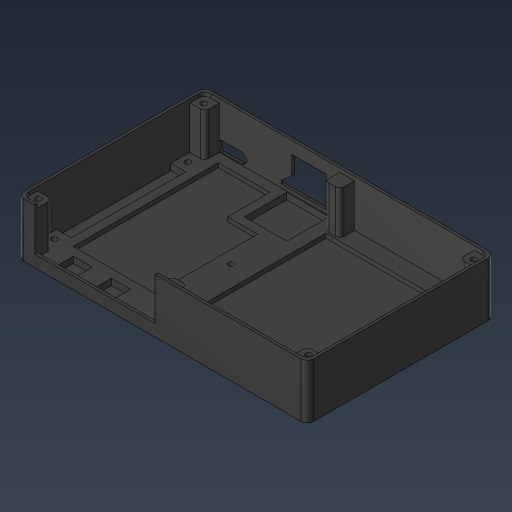
# Autodesk Inventor part: Gehaeuse BS v3
Saved by Autodesk Inventor 2023.1 (Build 271208000, 208)
## iProperties
Part Number: Gehaeuse BS v3
Material: PC/ABS-Kunststoff
Document SubType Name: Modeling
Designer: rYan
Density: 0.357273 g/cm^3
Appearance: Glatt - Schwarz
Mass: 15.1858 g
Surface Area: 455.446 cm^2
Volume: 42.5049 cm^3
Author: rYan
Autodesk Inventor part; units mm, degrees
ref_plane "YZ Plane" through (0, 0, 0) normal (1, 0, 0) x (0, 1, 0)
ref_plane "XZ Plane" through (0, 0, 0) normal (0, 1, 0) x (-1, 0, 0)
ref_plane "XY Plane" through (0, 0, 0) normal (0, 0, 1) x (1, 0, 0)
sketch "Skizze1" plane through (0, 0, 0) normal (0, 0, 1) x (1, 0, 0)
  line L0 (-68.45, -44.2) -> (68.45, -44.2)
  line L1 (68.45, -44.2) -> (68.45, 44.2)
  line L2 (68.45, 44.2) -> (-68.45, 44.2)
  line L3 (-68.45, 44.2) -> (-68.45, -44.2)
  line L4 (-68.45, -44.2) -> (68.45, 44.2) construction
  line L5 (68.45, -44.2) -> (-68.45, 44.2) construction
  circle A0 centre (-63.75, -39) radius 1.375
  circle A1 centre (63.75, -39) radius 1.375
  circle A2 centre (63.75, 39) radius 1.375
  circle A3 centre (-63.75, 39) radius 1.375
  line L6 (0, 61.88) -> (0, -61.88) projected
  line L7 (-95.83, 0) -> (95.83, 0) projected
  circle A4 centre (-63.75, 31.5) radius 1.375
  circle A5 centre (-63.75, -31.5) radius 1.375
  line L8 (-63.75, 39) -> (-63.75, 31.5) construction
  circle A6 centre (-11.75, 0) radius 1.375
  point P0 (0, 0)
  dimension "d0" = 136.9
  dimension "d1" = 88.4
  dimension "d2" = 2.75
  dimension "d3" = 127.5
  dimension "d4" = 78
  dimension "d7" = 63
  dimension "d8" = 2.75
  dimension "d9" = 2.75
  dimension "d10" = 52
  constraints: 14 end point, 7 centre point, 2 midpoint, 2 parallel, 1 horizontal, 1 perpendicular, 1 point on line, 1 vertical, 4 other
  measures "d0" distance of L2.end L1.end
  measures "d1" distance of L1.end L0.end
  measures "d2" diameter of A3
  measures "d3" distance of A1.centre A0.centre
  measures "d4" distance of A0.centre L8.start
  measures "d7" distance of A5.centre L8.end
  measures "d8" diameter of A4
  measures "d9" diameter of A6
  measures "d10" horizontal distance of A6.centre L8.end
extrude "Extrusion1" add sketch "Skizze1" along normal blind 3.6 contours L3 L7 A6 L6 L0 | L6 L7 L1 L0 | L3 L2 L6 L7 A6 | L6 L2 L1 L7
sketch "Skizze2" plane through (0, 0, 0) normal (0, 0, -1) x (-1, 0, 0)
  circle A0 centre (63.75, -31.5) radius 1.375 projected
  circle A1 centre (63.75, 31.5) radius 1.375 projected
  circle A2 centre (11.75, 0) radius 1.375 projected
  line L0 (67.05, -28.2) -> (60.45, -28.2)
  line L1 (60.45, -28.2) -> (60.45, -34.8)
  line L2 (60.45, -34.8) -> (67.05, -34.8)
  line L3 (67.05, -34.8) -> (67.05, -28.2)
  line L4 (67.05, -28.2) -> (60.45, -34.8) construction
  line L5 (60.45, -28.2) -> (67.05, -34.8) construction
  line L6 (67.05, 34.8) -> (60.45, 34.8)
  line L7 (60.45, 34.8) -> (60.45, 28.2)
  line L8 (60.45, 28.2) -> (67.05, 28.2)
  line L9 (67.05, 28.2) -> (67.05, 34.8)
  circle A3 centre (63.75, 31.5) radius 1.375 projected
  line L10 (67.05, 34.8) -> (60.45, 28.2) construction
  line L11 (60.45, 34.8) -> (67.05, 28.2) construction
  line L12 (15.05, 3.3) -> (8.45, 3.3)
  line L13 (8.45, 3.3) -> (8.45, -3.3)
  line L14 (8.45, -3.3) -> (15.05, -3.3)
  line L15 (15.05, -3.3) -> (15.05, 3.3)
  line L16 (15.05, 3.3) -> (8.45, -3.3) construction
  line L17 (8.45, 3.3) -> (15.05, -3.3) construction
  point P0 (0, 0)
  dimension "d11" = 6.6
  dimension "d12" = 6.6
  constraints: 36 end point, 6 midpoint, 6 parallel, 4 equal length, 3 horizontal, 3 perpendicular
  measures "d11" distance of L2.end L1.end
  measures "d12" distance of L1.end L0.end
extrude "Extrusion2" [suppressed]
sketch "Skizze3" plane through (0, 0, 3.6) normal (0, 0, 1) x (1, 0, 0)
  circle A0 centre (-63.75, 31.5) radius 1.375 projected
  circle A1 centre (-63.75, -31.5) radius 1.375 projected
  circle A2 centre (-11.75, 0) radius 1.375 projected
  line L0 (-63.75, 31.5) -> (-63.75, -31.5) construction
  line L1 (-95.83, 0) -> (95.83, 0) projected
  line L2 (-67.25, -27) -> (-60.25, -27)
  line L3 (-60.25, -27) -> (-60.25, 27)
  line L4 (-60.25, 27) -> (-67.25, 27)
  line L5 (-67.25, 27) -> (-67.25, -27)
  line L6 (-67.25, -27) -> (-60.25, 27) construction
  line L7 (-60.25, -27) -> (-67.25, 27) construction
  line L8 (-52.25, -34) -> (-43.25, -34)
  line L9 (-43.25, -34) -> (-43.25, -43)
  line L10 (-43.25, -43) -> (-52.25, -43)
  line L11 (-52.25, -43) -> (-52.25, -34)
  line L12 (-34.25, -34) -> (-25.25, -34)
  line L13 (-25.25, -34) -> (-25.25, -43)
  line L14 (-25.25, -43) -> (-34.25, -43)
  line L15 (-34.25, -43) -> (-34.25, -34)
  line L16 (-47.75, -34) -> (-47.75, -43) construction
  line L17 (-29.75, -34) -> (-29.75, -43) construction
  line L18 (-52.25, -38.5) -> (-43.25, -38.5) construction
  line L19 (-27.95, 22.5) -> (-7.95, 22.5)
  line L20 (-7.95, 22.5) -> (-7.95, 42.5)
  line L21 (-7.95, 42.5) -> (-27.95, 42.5)
  line L22 (-27.95, 42.5) -> (-27.95, 22.5)
  line L23 (-17.95, 42.5) -> (-17.95, 22.5) construction
  point P0 (0, 0)
  point P1 (-63.75, 0)
  dimension "d15" = 7
  dimension "d16" = 54
  dimension "d17" = 9
  dimension "d18" = 9
  dimension "d19" = 9
  dimension "d20" = 18
  dimension "d21" = 16
  dimension "d22" = 7
  dimension "d23" = 20
  dimension "d25" = 11
  dimension "d26" = 20
  dimension "d29" = 45.8
  constraints: 46 end point, 11 midpoint, 8 parallel, 4 horizontal, 4 perpendicular, 3 point on line, 1 vertical
  measures "d15" distance of L4.end L3.end
  measures "d16" distance of L3.end L2.end
  measures "d17" distance of L8.start L8.end
  measures "d18" distance of L12.start L12.end
  measures "d19" distance of L10.end L8.start
  measures "d20" distance between parallel lines of L17 L16
  measures "d21" distance between parallel lines of L16 L0
  measures "d22" distance from line of L18 L0.end
  measures "d23" distance of L19.start L19.end
  measures "d25" distance from line of L21 L0.start
  measures "d26" distance of L19.end L20.end
  measures "d29" distance between parallel lines of L23 L0
extrude "Extrusion3" cut sketch "Skizze3" against normal blind 3 contours L3 L2 L5 L1 | L1 L5 L4 L3 | L8 L9 L10 L11 | L12 L13 L14 L15 | L22 L21 L20 L19
sketch "Skizze4" plane through (0, 0, 3.6) normal (0, 0, 1) x (1, 0, 0)
  line L0 (-31.95, 18.5) -> (-17.75, 18.5)
  line L1 (-17.75, 18.5) -> (-17.75, -30)
  line L2 (-17.75, -30) -> (-56.25, -30)
  line L3 (-56.25, -30) -> (-56.25, 38.5)
  line L4 (-31.95, 18.5) -> (-31.95, 38.5)
  line L5 (-31.95, 38.5) -> (-56.25, 38.5)
  line L6 (-1.95, 35) -> (58.05, 35)
  line L7 (58.05, 35) -> (58.05, -35)
  line L8 (58.05, -35) -> (-1.95, -35)
  line L9 (-1.95, -35) -> (-1.95, 35)
  line L10 (-7.95, 22.5) -> (-27.95, 22.5) projected
  line L11 (-7.95, 42.5) -> (-7.95, 22.5) projected
  line L12 (-27.95, 42.5) -> (-7.95, 42.5) projected
  line L13 (-27.95, 22.5) -> (-27.95, 42.5) projected
  line L14 (-60.25, -27) -> (-67.25, -27) projected
  line L15 (-60.25, 27) -> (-60.25, -27) projected
  line L16 (-67.25, 27) -> (-60.25, 27) projected
  line L17 (-67.25, -27) -> (-67.25, 27) projected
  line L18 (-34.25, -34) -> (-25.25, -34) projected
  line L19 (-34.25, -43) -> (-34.25, -34) projected
  line L20 (-25.25, -43) -> (-34.25, -43) projected
  line L21 (-25.25, -34) -> (-25.25, -43) projected
  circle A0 centre (-11.75, 0) radius 1.375 projected
  line L22 (-95.83, 0) -> (95.83, 0) projected
  line L23 (0, 61.88) -> (0, -61.88) projected
  point P0 (0, 0)
  dimension "d30" = 4
  dimension "d31" = 4
  dimension "d32" = 4
  dimension "d34" = 4
  dimension "d35" = 6
  dimension "d36" = 4
  dimension "d37" = 6
  dimension "d38" = 70
  dimension "d39" = 60
  constraints: 20 end point, 4 parallel, 2 horizontal, 2 perpendicular, 1 other
  measures "d30" distance between parallel lines of L15 L3
  measures "d31" distance between parallel lines of L4 L13
  measures "d32" distance between parallel lines of L12 L5
  measures "d34" distance between parallel lines of L18 L2
  measures "d35" distance from line of L1 A0.centre
  measures "d36" distance between parallel lines of L10 L0
  measures "d37" distance between parallel lines of L11 L9
  measures "d38" distance of L6.end L7.end
  measures "d39" distance of L6.start L6.end
extrude "Extrusion4" cut sketch "Skizze4" against normal blind 2 contours L9 L6 L23 L22 | L22 L23 L8 L9 | L0 L1 L22 L3 L5 L4 | L1 L2 L3 L22 | L23 L6 L7 L22 | L22 L7 L8 L23
sketch "Skizze5" plane through (0, 0, 3.6) normal (0, 0, 1) x (1, 0, 0)
  circle A0 centre (-63.75, 39) radius 1.375 projected
  circle A1 centre (-63.75, -39) radius 1.375 projected
  circle A2 centre (63.75, -39) radius 1.375 projected
  circle A3 centre (63.75, 39) radius 1.375 projected
  line L0 (-67.25, 43) -> (-60.25, 43)
  line L1 (-60.25, 43) -> (-60.25, 36)
  line L2 (-60.25, 36) -> (-67.25, 36)
  line L3 (-67.25, 36) -> (-67.25, 43)
  line L4 (-67.25, -43) -> (-60.25, -43)
  line L5 (-60.25, -43) -> (-60.25, -36)
  line L6 (-60.25, -36) -> (-67.25, -36)
  line L7 (-67.25, -36) -> (-67.25, -43)
  line L8 (60.25, 36) -> (67.25, 36)
  line L9 (67.25, 36) -> (67.25, 43)
  line L10 (67.25, 43) -> (60.25, 43)
  line L11 (60.25, 43) -> (60.25, 36)
  circle A4 centre (63.75, 39) radius 1.375 projected
  line L12 (60.25, -43) -> (67.25, -43)
  line L13 (67.25, -43) -> (67.25, -36)
  line L14 (67.25, -36) -> (60.25, -36)
  line L15 (60.25, -36) -> (60.25, -43)
  line L16 (0, 61.88) -> (0, -61.88) projected
  line L17 (-95.83, 0) -> (95.83, 0) projected
  line L18 (-63.75, 36) -> (-63.75, 43) construction
  line L19 (3.5, -43) -> (-3.5, -43)
  line L20 (-3.5, -43) -> (-3.5, -36)
  line L21 (-3.5, -36) -> (3.5, -36)
  line L22 (3.5, -36) -> (3.5, -43)
  line L23 (3.5, 36) -> (-3.5, 36)
  line L24 (-3.5, 36) -> (-3.5, 43)
  line L25 (-3.5, 43) -> (3.5, 43)
  line L26 (3.5, 43) -> (3.5, 36)
  point P0 (0, 0)
  dimension "d42" = 7
  dimension "d46" = 3
  dimension "d47" = 4
  dimension "d51" = 7
  constraints: 50 end point, 12 parallel, 6 horizontal, 6 perpendicular, 4 collinear, 2 midpoint, 2 point on line, 14 other
  measures "d42" distance of L1.end L2.end
  measures "d46" distance from line of L2 A0.centre
  measures "d47" distance from line of L0 A0.centre
  measures "d51" distance of L19.start L19.end
extrude "Extrusion5" add sketch "Skizze5" along normal blind 20.2
sketch "Skizze7" plane through (0, 0, 23.8) normal (0, 0, 1) x (1, 0, 0)
  line L0 (-3.5, -43) -> (3.5, -43) projected
  line L1 (3.5, -43) -> (3.5, -36) projected
  line L2 (3.5, -36) -> (-3.5, -36) projected
  line L3 (-3.5, -36) -> (-3.5, -43) projected
  point P0 (0, 0)
extrude "Extrusion7" cut sketch "Skizze7" against normal blind 3.2
fillet "Rundung1" radius 2 8 edges at (-60.25, 36, 13.7) (-60.25, -36, 13.7) (60.25, 36, 13.7) (60.25, -36, 13.7) (3.5, -36, 12.1) (3.5, 36, 13.7) (-3.5, 36, 13.7) (-3.5, -36, 12.1)
sketch "Skizze6" plane through (0, 0, 3.6) normal (0, 0, 1) x (1, 0, 0)
  line L0 (-60.25, 43) -> (-67.25, 43) projected
  line L1 (-67.25, 43) -> (-67.25, 36) projected
  line L2 (67.25, -43) -> (67.25, -36) projected
  line L3 (60.25, -43) -> (67.25, -43) projected
  line L4 (-67.25, 43) -> (67.25, 43)
  line L5 (67.25, 43) -> (67.25, -43)
  line L6 (67.25, -43) -> (-67.25, -43)
  line L7 (-67.25, -43) -> (-67.25, 43)
  line L8 (68.45, 44.2) -> (-68.45, 44.2)
  line L9 (-68.45, 44.2) -> (-68.45, -44.2)
  line L10 (-68.45, -44.2) -> (68.45, -44.2)
  line L11 (68.45, -44.2) -> (68.45, 44.2)
  point P0 (0, 0)
  dimension "d48" = 1.2
  constraints: 16 end point, 4 parallel, 2 perpendicular, 1 horizontal, 3 other
  measures "d48" distance between parallel lines of L4 L8
extrude "Extrusion6" add sketch "Skizze6" along normal blind 22
sketch "Skizze8" plane through (-68.45, 44.2, 0) normal (0, 1, 0) x (1, 0, 0)
  line L0 (68.45, 3.96) -> (68.45, -23.76) projected
  line L1 (164.28, 0) -> (-27.38, 0) projected
  line L2 (19.2, -4) -> (8.2, -4)
  line L3 (8.2, -4) -> (8.2, -9)
  line L4 (8.2, -9) -> (19.2, -9)
  line L5 (19.2, -9) -> (19.2, -4)
  line L6 (19.2, -4) -> (8.2, -9) construction
  line L7 (8.2, -4) -> (19.2, -9) construction
  line L8 (58.55, -5.2) -> (42.35, -5.2)
  line L9 (42.35, -5.2) -> (42.35, -19.8)
  line L10 (42.35, -19.8) -> (58.55, -19.8)
  line L11 (58.55, -19.8) -> (58.55, -5.2)
  line L12 (58.55, -5.2) -> (42.35, -19.8) construction
  line L13 (42.35, -5.2) -> (58.55, -19.8) construction
  line L14 (42.35, -5.2) -> (37.35, -5.2)
  line L15 (37.35, -5.2) -> (37.35, -6.7)
  line L16 (37.35, -6.7) -> (42.35, -10.8955)
  line L17 (19.2, -9) -> (21.7, -6.5)
  line L18 (21.7, -6.5) -> (19.2, -4)
  line L19 (21.7, -6.5) -> (13.7, -6.5) construction
  point P0 (68.45, 0)
  point P1 (50.45, -12.5)
  dimension "d55" = 54.75
  dimension "d56" = 6.5
  dimension "d57" = 11
  dimension "d58" = 5
  dimension "d61" = 18
  dimension "d63" = 14.6
  dimension "d64" = 16.2
  dimension "d65" = 5.2
  dimension "d66" = 50
  dimension "d67" = 1.5
  dimension "d68" = 5
  dimension "d69" = 2.5
  constraints: 36 end point, 4 horizontal, 4 midpoint, 4 parallel, 3 perpendicular, 3 point on line, 1 vertical, 1 other
  measures "d55" distance from line of L0 L19.end
  measures "d56" distance from line of L1 L19.end
  measures "d57" distance of L3.end L4.end
  measures "d58" distance of L4.end L2.start
  measures "d61" distance from line of L0 point (50.45, -12.5)
  measures "d63" distance of L10.end L8.start
  measures "d64" distance of L9.end L10.end
  measures "d65" distance between parallel lines of L8 L1
  measures "d66" angle of L16 L15
  measures "d67" distance of L14.end L15.end
  measures "d68" distance of L8.end L14.end
  measures "d69" distance from line of L5 L17.end
extrude "Extrusion8" cut sketch "Skizze8" against normal up to surface (1.2 mm away)
sketch "Skizze9" plane through (-68.45, -44.2, 0) normal (0, -1, 0) x (1, 0, 0)
  line L0 (0, 0) -> (136.9, 0) projected
  line L1 (136.9, 0) -> (136.9, 25.6) projected
  line L2 (0, 25.6) -> (136.9, 25.6) projected
  line L3 (0, 0) -> (0, 25.6) projected
  line L4 (135.7, 25.6) -> (1.2, 25.6) projected
  line L5 (8.2, 25.6) -> (64.95, 25.6)
  line L6 (64.95, 25.6) -> (64.95, 5.6)
  line L7 (64.95, 5.6) -> (8.2, 5.6)
  line L8 (8.2, 5.6) -> (8.2, 25.6)
  line L9 (16.2, 3.6) -> (25.2, 3.6) projected
  line L10 (16.2, 3.6) -> (16.2, 0.6) projected
  line L11 (16.2, 0.6) -> (25.2, 0.6) projected
  line L12 (25.2, 3.6) -> (25.2, 0.6) projected
  line L13 (34.2, 3.6) -> (43.2, 3.6) projected
  line L14 (34.2, 3.6) -> (34.2, 0.6) projected
  line L15 (34.2, 0.6) -> (43.2, 0.6) projected
  line L16 (43.2, 3.6) -> (43.2, 0.6) projected
  line L17 (16.2, 0.6) -> (25.2, 0.6) construction
  line L18 (20.7, 0.6) -> (20.7, 3.6) construction
  line L19 (34.2, 0.6) -> (43.2, 0.6) construction
  line L20 (38.7, 0.6) -> (38.7, 3.6) construction
  line L21 (8.2, 23.8) -> (8.2, 3.6) projected
  line L22 (8.2, 3.6) -> (8.2, 23.8) projected
  point P0 (68.45, 0)
  dimension "d73" = 64.95
  dimension "d75" = 2
  constraints: 12 end point, 4 midpoint, 1 collinear, 1 horizontal, 1 parallel, 1 perpendicular, 1 point on line
  measures "d73" distance between parallel lines of L3 L6
  measures "d75" distance between parallel lines of L7 L9
extrude "Extrusion9" cut sketch "Skizze9" against normal up to surface (1.2 mm away) contours L2 L6 L7 L8
fillet "Rundung2" radius 3 8 edges at (-68.45, -44.2, 12.8) (-68.45, 44.2, 12.8) (68.45, -44.2, 12.8) (68.45, 44.2, 12.8) (67.25, 43, 24.7) (67.25, -43, 24.7) (-67.25, -43, 24.7) (-67.25, 43, 24.7)
fillet "Rundung3" radius 1 6 edges at (-26.1, 43.6, 10.8955) (-49.25, 43.6, 9) (-49.25, 43.6, 4) (-46.75, 43.6, 6.5) (-60.25, 43.6, 9) (-60.25, 43.6, 4)
equation "\"d9\" = d8"
equation "\"d18\" = d17"
equation "\"d51\" = d42"
